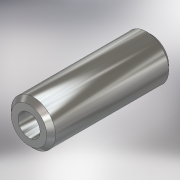
# Autodesk Inventor part: Piston pin
Saved by Autodesk Inventor 2019 (Build 230136000, 136)
## iProperties
Created: 2020-05-28
Part Number: Piston pin
Material: Generic
Document SubType Name: Modeling
Designer: Manoj
Density: 1 g/cm^3
Appearance: Chrome - Polished
Author: Manoj
Autodesk Inventor part; units mm, degrees
ref_plane "YZ Plane" through (0, 0, 0) normal (1, 0, 0) x (0, 1, 0)
ref_plane "XZ Plane" through (0, 0, 0) normal (0, 1, 0) x (-1, 0, 0)
ref_plane "XY Plane" through (0, 0, 0) normal (0, 0, 1) x (1, 0, 0)
sketch "Sketch1" plane through (0, 0, 0) normal (0, 0, 1) x (1, 0, 0)
  circle A0 centre (0, 0) radius 6.35
  circle A1 centre (0, 0) radius 12.7
  dimension "d0" = 12.7
  dimension "d1" = 25.4
  constraints: 2 centre point, 2 coincident
  measures "d0" diameter of A0
  measures "d1" diameter of A1
extrude "Extrusion1" add sketch "Sketch1" along normal mid plane 69.85
chamfer "Chamfer1" distance 2.5 angle 45 1 edges at (-12.7, 0, -34.925) measured on face at (10.3988, -1.5197, -34.925)
chamfer "Chamfer2" distance 2.5 angle 45 1 edges at (-12.7, 0, 34.925) measured on face at (10.3988, -1.5197, 34.925)
body "Solid1"
